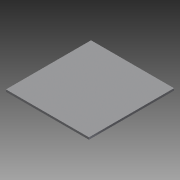
# Autodesk Inventor part: Middle
Saved by Autodesk Inventor 2015 (Build 190159000, 159)
## iProperties
Created: 2016-03-23
Part Number: Middle
Material: Generic
Document SubType Name: Modeling
Designer: Noah
Density: 1 g/cm^3
Appearance: Denim - Blue
Author: Noah
Autodesk Inventor part; units mm, degrees
ref_plane "YZ Plane" through (0, 0, 0) normal (1, 0, 0) x (0, 1, 0)
ref_plane "XZ Plane" through (0, 0, 0) normal (0, 1, 0) x (-1, 0, 0)
ref_plane "XY Plane" through (0, 0, 0) normal (0, 0, 1) x (1, 0, 0)
sketch "Sketch1" plane through (0, 0, 0) normal (0, 0, 1) x (1, 0, 0)
  line L0 (-164, 172) -> (172, 172)
  line L1 (172, 172) -> (172, -142)
  line L2 (172, -142) -> (-164, -142)
  line L3 (-164, -142) -> (-164, 172)
  point P0 (0, 0)
  dimension "d0" = 336
  dimension "d1" = 314
  dimension "d2" = 172
  dimension "d3" = 172
  constraints: 8 end point, 2 parallel, 1 horizontal, 1 perpendicular
  measures "d0" distance of L0.start L0.end
  measures "d1" distance of L0.end L1.end
  measures "d2" distance from line of L0 point (0, 0)
  measures "d3" distance from line of L1 point (0, 0)
extrude "Extrusion1" add sketch "Sketch1" along normal blind 8
equation "\"d0\" = -2 * wall_width + edge_length - wall_width_small"
equation "\"d2\" = -wall_width + 0.5 * edge_length"
equation "\"d3\" = -wall_width + 0.5 * edge_length"
equation "\"d4\" = wall_width_small"
equation "\"wall_width\" = 8"
equation "\"edge_length\" = 360"
equation "\"wall_width_small\" = 8"
body "Solid1"
